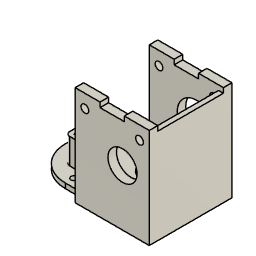
Potentionmeter_Bot (Autodesk Fusion 360 design; units mm, degrees)
Autodesk Fusion 360 part; units mm, degrees
note: some values were not read from the file. Set by a fixed rule: which face or edge a step refers to.
sketch "スケッチ1" plane through (0, 0, 0) normal (0, 0, 1) x (1, 0, 0)
  line L0 (5, -5) -> (-5, -5)
  line L1 (-5, -5) -> (-5, 5)
  line L2 (-5, 5) -> (5, 5)
  line L3 (5, 5) -> (5, -5)
  line L4 (5, -5) -> (-5, 5) construction
  line L5 (-5, -5) -> (5, 5) construction
  line L6 (7, -7) -> (-7, -7)
  line L7 (-7, -7) -> (-7, 7)
  line L8 (-7, 7) -> (7, 7)
  line L9 (7, 7) -> (7, -7)
  line L10 (7, -7) -> (-7, 7) construction
  line L11 (-7, -7) -> (7, 7) construction
  dimension "d1" = 10
  dimension "d2" = 10
  dimension "d3" = 14
  dimension "d4" = 14
  constraint horizontal L0
  constraint perpendicular L0 L1
  constraint parallel L0 L2
  constraint parallel L1 L3
  constraint coincident L4 origin
  constraint coincident L5 origin
  constraint horizontal L6
  constraint perpendicular L6 L7
  constraint parallel L6 L8
  constraint parallel L7 L9
  constraint coincident L10 origin
  constraint coincident L11 origin
  measures "d1" distance of L1.end L2.end
  measures "d2" distance of L0.end L1.end
  measures "d3" distance of L7.end L8.end
  measures "d4" distance of L6.end L7.end
extrude "押し出し1" add sketch "スケッチ1" along normal blind 8 contours L6 L7 L8 L9 picked at (-6.333333, 1.666667) makes body 1
sketch "スケッチ2" plane through (0, 0, 0) normal (0, 0, -1) x (1, 0, 0)
  line L0 (5, -5) -> (-5, -5)
  line L1 (-5, -5) -> (-5, 5)
  line L2 (-5, 5) -> (5, 5)
  line L3 (5, 5) -> (5, -5)
  line L4 (-7, -7) -> (7, -7)
  line L5 (7, -7) -> (7, 7)
  line L6 (7, 7) -> (-7, 7)
  line L7 (-7, 7) -> (-7, -7)
  circle A0 centre (0, 7) radius 7
  circle A1 centre (0, -7) radius 7
  circle A2 centre (7, 0) radius 7
  circle A3 centre (-7, 0) radius 7
  constraint midpoint L6 A0.centre
  constraint coincident L5.end A0
  constraint midpoint L4 A1.centre
  constraint coincident L4.end A1
  constraint midpoint L5 A2.centre
  constraint coincident L4.end A2
  constraint midpoint L7 A3.centre
  constraint coincident L4.start A3
extrude "押し出し2" add sketch "スケッチ2" against normal blind 2 contours L4 A1 | L5 A2 | L7 A3 | L6 A0 picked at (0.519216, -9.274832) picked at (8.528008, 1.763416) picked at (-9.326809, -0.17437) picked at (-0.17437, 9.326809) bodies 1
cylinder "円柱プリミティブ1" cut diameter 2.5 height -14 placed x (0, 0, -1) y (0, 1, 0) z (1, 0, 0) at (7, 0, 5) bodies 1
sketch "スケッチ4" plane through (0, 0, 2) normal (0, 0, 1) x (-1, 0, 0)
  arc A0 (7, 7) -> (-7, 7) centre (0, 7) ccw
  line L0 (-7, 7) -> (7, 7)
  line L1 (0, 7) -> (0, 14)
  circle A1 centre (0, 10.5) radius 1.25
  dimension "d11" = 2.5
  constraint coincident A0.centre L1.start
  constraint midpoint A0 L1.end
  constraint midpoint L1 A1.centre
  measures "d11" diameter of A1
sketch "スケッチ5" plane through (0, 0, 2) normal (0, 0, 1) x (-1, 0, 0)
  arc A0 (7, -7) -> (7, 7) centre (7, 0) ccw
  line L0 (7, 7) -> (7, -7)
  line L1 (7, 0) -> (14, 0)
  circle A1 centre (10.5, 0) radius 1.25
  dimension "d12" = 2.5
  constraint coincident A0.centre L1.start
  constraint midpoint A0 L1.end
  constraint midpoint L1 A1.centre
  measures "d12" diameter of A1
sketch "スケッチ6" plane through (0, 0, 2) normal (0, 0, 1) x (-1, 0, 0)
  arc A0 (-7, -7) -> (7, -7) centre (0, -7) ccw
  line L0 (7, -7) -> (-7, -7)
  line L1 (0, -7) -> (0, -14)
  circle A1 centre (0, -10.5) radius 1.25
  dimension "d13" = 2.5
  constraint coincident A0.centre L1.start
  constraint midpoint A0 L1.end
  constraint midpoint L1 A1.centre
  measures "d13" diameter of A1
sketch "スケッチ7" plane through (0, 0, 2) normal (0, 0, 1) x (-1, 0, 0)
  arc A0 (-7, 7) -> (-7, -7) centre (-7, 0) ccw
  line L0 (-7, -7) -> (-7, 7)
  line L1 (-7, 0) -> (-14, 0)
  circle A1 centre (-10.5, 0) radius 1.25
  dimension "d14" = 2.5
  constraint coincident A0.centre L1.start
  constraint midpoint A0 L1.end
  constraint midpoint L1 A1.centre
  measures "d14" diameter of A1
extrude "押し出し3" cut sketch "スケッチ4" sketch "スケッチ7" sketch "スケッチ6" sketch "スケッチ5" against normal blind 2 contours L1 A1 | L1 A1 picked at (0.272859, 10.814896) picked at (-0.448578, 10.258724) of sketch 2 contours L1 A1 | L1 A1 picked at (-10.25407, 0.510679) picked at (-10.083333, -0.651526) of sketch 3 contours L1 A1 | L1 A1 picked at (-0.644249, -10.180438) picked at (0.17309, -10.120987) of sketch 4 contours L1 A1 | L1 A1 picked at (10.916667, -0.651526) picked at (10.741276, 0.448578) bodies 1
extrude "押し出し4" cut 1 faces at (7.75, 0, 2) along direction (0, 0, -1) blind 2 on bodies 1 bodies 1
sketch "スケッチ8" plane through (0, 0, 0) normal (0, 0, -1) x (1, 0, 0)
  line L0 (7, -7) -> (7, 7)
  arc A0 (7, 7) -> (-7, 7) centre (0, 7) ccw
  arc A1 (-7, 7) -> (-7, -7) centre (-7, 0) ccw
  arc A2 (-7, -7) -> (7, -7) centre (0, -7) ccw
  line L1 (5, -5) -> (-5, -5)
  line L2 (-5, -5) -> (-5, 5)
  line L3 (-5, 5) -> (5, 5)
  line L4 (5, 5) -> (5, -5)
  circle A3 centre (-10.5, 0) radius 1.25
  circle A4 centre (0, 10.5) radius 1.25
  circle A5 centre (0, -10.5) radius 1.25
  line L5 (-10.5, 0) -> (26.5, 0)
  line L6 (26.5, -5) -> (-10.5, -5)
  line L7 (-10.5, -5) -> (-10.5, 5)
  line L8 (-10.5, 5) -> (26.5, 5)
  line L9 (26.5, 5) -> (26.5, -5)
  line L10 (26.5, -5) -> (-10.5, 5) construction
  line L11 (-10.5, -5) -> (26.5, 5) construction
  circle A6 centre (26.5, 0) radius 8
  line L12 (26.5, 5) -> (26.5, 8)
  line L13 (18.5, 0) -> (18.5, 8)
  line L14 (18.5, 8) -> (26.5, 8)
  line L15 (18.5, 0) -> (18.5, -8)
  line L16 (26.5, -5) -> (26.5, -8)
  line L17 (26.5, -8) -> (18.5, -8)
  line L18 (18.5, -8) -> (14.5, -8)
  line L19 (18.5, 8) -> (14.5, 8)
  line L20 (14.5, -8) -> (14.5, 8)
  point P0 (8, 0)
  dimension "d19" = 37
  dimension "d20" = 37
  dimension "d21" = 10
  dimension "d22" = 16
  dimension "d27" = 4
  dimension "d28" = 4
  constraint coincident A3.centre L5.start
  constraint perpendicular L0 L5
  constraint horizontal L6
  constraint perpendicular L6 L7
  constraint parallel L6 L8
  constraint parallel L7 L9
  constraint coincident L10 P0
  constraint coincident L11 P0
  constraint midpoint L5 P0
  constraint coincident L5.end A6.centre
  constraint coincident A6 L12.end
  constraint perpendicular L8 L12
  constraint coincident L5 L13.start
  constraint coincident A6 L13.start
  constraint tangent A6 L13
  constraint perpendicular L13 L14
  constraint tangent A6 L15
  constraint coincident A6 L16.end
  constraint perpendicular L6 L16
  constraint perpendicular L15 L17
  constraint perpendicular L15 L18
  constraint perpendicular L13 L19
  measures "d19" distance of A3.centre L5.end
  measures "d20" distance of L7.end L8.end
  measures "d21" distance of L6.end L7.end
  measures "d22" diameter of A6
  measures "d27" distance of L15.end L18.end
  measures "d28" distance of L13.end L19.end
extrude "押し出し5" add sketch "スケッチ8" against normal blind 11 separate body contours L5 L6 L15 L20 | L6 L15 L18 L20 | L5 L8 L13 L20 | L6 A6 L15 | L6 A6 L15 L17 | L8 L13 L19 L20 | L8 A6 L13 | L8 A6 L13 L14 picked at (15.833333, -1.666667) picked at (15.833333, -6) picked at (15.833333, 1.666667) picked at (19.464588, -4.704603) picked at (19.085001, -6) picked at (17.166667, 6) picked at (19.464588, 4.704603) picked at (19.085001, 6) makes body 2
extrude "押し出し6" add sketch "スケッチ8" against normal blind 2 contours L0 L5 L6 L20 | L0 L5 L8 L20 | L5 L6 L15 L20 | L5 L8 L13 L20 picked at (9.5, -3.333333) picked at (9.5, 3.333333) picked at (15.833333, -1.666667) picked at (15.833333, 1.666667) bodies 1 2
sketch "スケッチ9" plane through (0, 0, 11) normal (0, 0, 1) x (-1, 0, 0)
  line L0 (-14.5, 8) -> (-26.5, 8)
  arc A0 (-26.5, -8) -> (-26.5, 8) centre (-26.5, 0) ccw
  line L1 (-26.5, -8) -> (-14.5, -8)
  line L2 (-14.5, -8) -> (-14.5, 8)
  line L3 (-26.5, 0) -> (-18.5, 0)
  line L4 (-22.5, 0) -> (-22.5, -8)
  line L5 (-22.5, 0) -> (-22.5, 8)
  constraint coincident A0.centre L3.start
  constraint midpoint A0 L3.end
  constraint midpoint L3 L4.start
  constraint coincident L1 L4.end
  constraint perpendicular L1 L4
  constraint coincident L0 L5.end
  constraint perpendicular L0 L5
extrude "押し出し7" cut sketch "スケッチ9" against normal blind 11 contours L0 A0 L5 | A0 L1 L4 picked at (-22.812844, 7.439747) picked at (-22.812844, -7.439747) bodies 1
extrude "押し出し8" add 1 faces at (7, 4.415502, 5.031138) along direction (1, 0, 0) blind 7.5 on bodies 1 bodies 1
extrude "押し出し9" cut 1 faces at (19.833333, -8, 3.666667) along direction (0, 1, 0) blind 1 on bodies 1 bodies 1
extrude "押し出し10" cut 1 faces at (19.833334, 8, 3.666667) along direction (0, -1, 0) blind 1 on bodies 1 bodies 1
sketch "スケッチ10" plane through (0, 0, 11) normal (0, 0, 1) x (-1, 0, 0)
  line L0 (-22.5, -7) -> (-14.5, -7)
  line L1 (-14.5, -7) -> (-14.5, 7)
  line L2 (-14.5, 7) -> (-22.5, 7)
  line L3 (-22.5, 7) -> (-22.5, 6.928203)
  arc A0 (-22.5, -6.928203) -> (-22.5, 6.928203) centre (-26.5, 0) ccw
  line L4 (-22.5, -6.928203) -> (-22.5, -7)
  line L5 (-22.5, -6.928203) -> (-22.5, 6.928203)
  circle A1 centre (-26.5, 0) radius 8.25
  dimension "d37" = 16.5
  constraint concentric A0 A1
  measures "d37" diameter of A1
extrude "押し出し11" cut sketch "スケッチ10" against normal blind 11 contours L0 L2 L3 A0 L4 A1 picked at (-22.048673, -6.727619) bodies 1
extrude "押し出し12" add 1 faces at (14.5, 2.333333, 10) along direction (-1, 0, 0) blind 7.5 on bodies 1 bodies 1
sketch "スケッチ11" plane through (0, -7, 0) normal (0, -1, 0) x (1, 0, 0)
  line L0 (22.133938, 0) -> (22.133938, 11)
  line L1 (22.133938, 11) -> (7, 11)
  line L2 (7, 11) -> (7, 8)
  line L3 (7, 8) -> (-7, 8)
  line L4 (-7, 8) -> (-7, 2)
  line L5 (-7, 2) -> (7, 2)
  line L6 (7, 2) -> (7, 0)
  line L7 (7, 0) -> (22.133938, 0)
  line L8 (7, 11) -> (7, 0)
  constraint coincident L1.end L2.start
  constraint coincident L6.end L7.start
extrude "押し出し13" add sketch "スケッチ11" along normal blind 8 contours L0 L1 L2 L6 L7 L8 picked at (17.089292, 6.333333) bodies 1
sketch "スケッチ12" plane through (0, 7, 0) normal (0, 1, 0) x (-1, 0, 0)
  line L0 (-22.133938, 11) -> (-22.133938, 0)
  line L1 (-22.133938, 0) -> (-7, 0)
  line L2 (-7, 0) -> (-7, 2)
  line L3 (-7, 2) -> (7, 2)
  line L4 (7, 2) -> (7, 8)
  line L5 (7, 8) -> (-7, 8)
  line L6 (-7, 8) -> (-7, 11)
  line L7 (-7, 11) -> (-22.133938, 11)
  line L8 (-7, 11) -> (-7, 0)
  constraint coincident L6.end L7.start
  constraint coincident L1.end L2.start
extrude "押し出し14" add sketch "スケッチ12" along normal blind 8 contours L0 L1 L2 L6 L7 L8 picked at (-17.089292, 6.333333) bodies 1
sketch "スケッチ13" plane through (0, 0, 11) normal (0, 0, 1) x (-1, 0, 0)
  arc A0 (-22.133938, -7) -> (-22.133938, 7) centre (-26.5, 0) ccw
  line L0 (-22.133938, -7) -> (-22.133938, -15)
  line L1 (-22.133938, -15) -> (-7, -15)
  line L2 (-7, -15) -> (-7, 15)
  line L3 (-7, 15) -> (-22.133938, 15)
  line L4 (-22.133938, 15) -> (-22.133938, 7)
  circle A1 centre (-26.5, 0) radius 8.25
  line L5 (-26.5, 0) -> (-22.133938, 0)
  line L6 (-22.133938, 0) -> (-22.133938, -15)
  line L7 (-22.133938, -15) -> (-26.5, -15)
  line L8 (-26.5, -15) -> (-26.5, 0)
  line L9 (-26.5, 0) -> (-22.133938, 0)
  line L10 (-22.133938, 0) -> (-22.133938, 15)
  line L11 (-22.133938, 15) -> (-26.5, 15)
  line L12 (-26.5, 15) -> (-26.5, 0)
  constraint concentric A0 A1
  constraint horizontal L5
  constraint vertical L6
  constraint horizontal L7
  constraint vertical L8
  constraint coincident A0.centre A1.centre
  constraint horizontal L9
  constraint vertical L10
  constraint horizontal L11
  constraint vertical L12
extrude "押し出し15" add sketch "スケッチ13" against normal blind 11 contours L0 A1 L6 L7 L8 | L4 A1 L10 L11 L12 picked at (-24.662481, -12.723316) picked at (-24.662481, 12.723316) bodies 1
sketch "スケッチ14" plane through (0, 0, 11) normal (0, 0, 1) x (-1, 0, 0)
  arc A0 (-26.5, -8.25) -> (-26.5, 8.25) centre (-26.5, 0) ccw
  line L0 (-26.5, -8.25) -> (-26.5, -15)
  line L1 (-26.5, -15) -> (-7, -15)
  line L2 (-7, -15) -> (-7, 15)
  line L3 (-7, 15) -> (-26.5, 15)
  line L4 (-26.5, 15) -> (-26.5, 8.25)
  line L5 (-7, 15) -> (-26.5, 15)
  line L6 (-26.5, 15) -> (-26.5, 17)
  line L7 (-26.5, 17) -> (-7, 17)
  line L8 (-7, 17) -> (-7, 15)
  line L9 (-7, -15) -> (-26.5, -15)
  line L10 (-26.5, -15) -> (-26.5, -17)
  line L11 (-26.5, -17) -> (-7, -17)
  line L12 (-7, -17) -> (-7, -15)
  dimension "d48" = 2
  dimension "d49" = 2
  constraint horizontal L5
  constraint vertical L6
  constraint horizontal L7
  constraint vertical L8
  constraint coincident L2.end L3.start
  constraint horizontal L9
  constraint vertical L10
  constraint horizontal L11
  constraint vertical L12
  constraint coincident L1.end L2.start
  measures "d48" distance of L2.end L7.end
  measures "d49" distance of L1.end L11.end
extrude "押し出し16" add sketch "スケッチ14" along normal blind 2 separate body contours L1 L9 L10 L11 L12 | L3 L5 L6 L7 L8 picked at (-20, -16.333333) picked at (-20, 15.666667) makes body 3 at (20, 15, 11.666667) makes body 4 at (20, -17, 11.666667)
extrude "押し出し17" add 2 faces at (20, -15.666667, 11) (20, 16.333333, 11) along direction (0, 0, -1) blind 11 on bodies 3 4 bodies 1 4 3
extrude "押し出し18" add 1 faces at (20, -15.666667, 13) along direction (0, 0, 1) blind 28 on bodies 1 bodies 1
extrude "押し出し19" add 1 faces at (26.5, -13.416667, 3.666667) along direction (1, 0, 0) blind 11 on bodies 1 bodies 1
extrude "押し出し20" add 1 faces at (26.5, 13.416667, 3.666667) along direction (1, 0, 0) blind 11 on bodies 1 bodies 1
sketch "スケッチ15" plane through (0, -15, 0) normal (0, 1, 0) x (-1, 0, 0)
  line L0 (-37.5, 11) -> (-7, 11)
  line L1 (-7, 11) -> (-7, 41)
  line L2 (-7, 41) -> (-37.5, 41)
  line L3 (-7, 11) -> (-26.5, 11)
  line L4 (-26.5, 11) -> (-26.5, 23)
  line L5 (-26.5, 23) -> (-7, 23)
  line L6 (-7, 23) -> (-7, 11)
  circle A0 centre (-26.5, 23) radius 6
  line L7 (-37.5, 41) -> (-37.5, 11)
  line L8 (-37.5, 11) -> (-7, 11)
  line L9 (-7, 11) -> (-7, 41)
  line L10 (-7, 41) -> (-37.5, 41)
  line L11 (-37.5, 41) -> (-37.5, 11)
  line L12 (-7, 41) -> (-11, 41)
  line L13 (-11, 41) -> (-11, 35.5)
  line L14 (-11, 35.5) -> (-7, 35.5)
  line L15 (-7, 35.5) -> (-7, 41)
  line L16 (-37.5, 41) -> (-33.5, 41)
  line L17 (-33.5, 41) -> (-33.5, 35.5)
  line L18 (-33.5, 35.5) -> (-37.5, 35.5)
  line L19 (-37.5, 35.5) -> (-37.5, 41)
  circle A1 centre (-33.5, 35.5) radius 1.6
  circle A2 centre (-11, 35.5) radius 1.6
  dimension "d56" = 19.5
  dimension "d57" = 12
  dimension "d58" = 12
  dimension "d63" = 4
  dimension "d64" = 5.5
  dimension "d65" = 4
  dimension "d66" = 5.5
  dimension "d67" = 3.2
  dimension "d68" = 3.2
  constraint horizontal L3
  constraint vertical L4
  constraint horizontal L5
  constraint vertical L6
  constraint coincident L0.end L1.start
  constraint coincident L4.end L5.start
  constraint horizontal L12
  constraint vertical L13
  constraint horizontal L14
  constraint vertical L15
  constraint coincident L1.end L2.start
  constraint horizontal L16
  constraint vertical L17
  constraint horizontal L18
  constraint vertical L19
  constraint coincident L2.end L7.start
  constraint coincident L17.end L18.start
  constraint coincident L13.end L14.start
  measures "d56" distance of L0.end L3.end
  measures "d57" distance of L0.end L5.end
  measures "d58" diameter of A0
  measures "d63" distance of L1.end L12.end
  measures "d64" distance of L1.end L14.end
  measures "d65" distance of L2.end L16.end
  measures "d66" distance of L2.end L18.end
  measures "d67" diameter of A1
  measures "d68" diameter of A2
extrude "押し出し21" cut sketch "スケッチ15" against normal blind 2 contours L4 L5 A0 | L4 L5 A0 | L17 L18 A1 | L17 L18 A1 | L13 L14 A2 | L13 L14 A2 picked at (-24.706428, 26.563216) picked at (-22.520357, 22.71537) picked at (-34.351735, 36.137601) picked at (-34.56071, 35.420511) picked at (-9.939106, 35.421744) picked at (-10.066194, 36.009896) bodies 1
sketch "スケッチ16" plane through (0, 0, 11) normal (0, 0, 1) x (-1, 0, 0)
  arc A0 (-26.5, -8.25) -> (-26.5, 8.25) centre (-26.5, 0) ccw
  line L0 (-26.5, -8.25) -> (-37.5, -8.25)
  line L1 (-37.5, -8.25) -> (-37.5, -15)
  line L2 (-37.5, -15) -> (-7, -15)
  line L3 (-7, -15) -> (-7, 15)
  line L4 (-7, 15) -> (-37.5, 15)
  line L5 (-37.5, 15) -> (-37.5, 8.25)
  line L6 (-37.5, 8.25) -> (-26.5, 8.25)
  circle A1 centre (-26.5, 0) radius 8.25
  line L7 (-37.5, -8.25) -> (-37.5, 8.25)
  constraint concentric A0 A1
  constraint coincident L0.end L1.start
  constraint coincident L5.end L6.start
extrude "押し出し22" add sketch "スケッチ16" against normal blind 11 contours L0 L6 A1 L7 picked at (-36.575644, 0.205508) bodies 1
extrude "押し出し23" add 1 faces at (14.5, -0.095795, 5.342047) along direction (-1, 0, 0) blind 9.5 on bodies 1 bodies 1
sketch "スケッチ17" plane through (0, 0, 8) normal (0, 0, 1) x (-1, 0, 0)
  line L0 (-7, 7) -> (-7, -7)
  line L1 (-7, -7) -> (7, -7)
  line L2 (7, -7) -> (7, 7)
  line L3 (7, 7) -> (-7, 7)
  line L4 (5, -5) -> (-5, -5)
  line L5 (-5, -5) -> (-5, 5)
  line L6 (-5, 5) -> (5, 5)
  line L7 (5, 5) -> (5, -5)
  line L8 (-5.25, 5.25) -> (5.25, 5.25)
  line L9 (5.25, 5.25) -> (5.25, -5.25)
  line L10 (5.25, -5.25) -> (-5.25, -5.25)
  line L11 (-5.25, -5.25) -> (-5.25, 5.25)
  line L12 (-5.25, 5.25) -> (5.25, -5.25) construction
  line L13 (5.25, 5.25) -> (-5.25, -5.25) construction
  dimension "d75" = 10.5
  dimension "d76" = 10.5
  constraint horizontal L8
  constraint perpendicular L8 L9
  constraint parallel L8 L10
  constraint parallel L9 L11
  constraint coincident L12 origin
  constraint coincident L13 origin
  measures "d75" distance of L9.end L10.end
  measures "d76" distance of L8.end L9.end
extrude "押し出し24" cut sketch "スケッチ17" against normal blind 8 contours L8 L9 L10 L11 picked at (1.666667, -5.166667) bodies 1
extrude "押し出し25" add 1 faces at (6.416667, -1.75, 8) along direction (0, 0, 1) blind 3 on bodies 1 bodies 1
sketch "スケッチ18" plane through (0, 0, 0) normal (0, 0, -1) x (1, 0, 0)
  line L0 (-5.25, -5.25) -> (-5.25, 5.25)
  line L1 (-5.25, 5.25) -> (5.25, 5.25)
  line L2 (5.25, 5.25) -> (5.25, -5.25)
  line L3 (5.25, -5.25) -> (-5.25, -5.25)
  line L4 (37.5, -17) -> (37.5, 17)
  line L5 (37.5, 17) -> (7, 17)
  line L6 (7, 17) -> (7, 7)
  arc A0 (7, 7) -> (-7, 7) centre (0, 7) ccw
  arc A1 (-7, 7) -> (-7, -7) centre (-7, 0) ccw
  arc A2 (-7, -7) -> (7, -7) centre (0, -7) ccw
  line L7 (7, -7) -> (7, -17)
  line L8 (7, -17) -> (37.5, -17)
  circle A3 centre (26.5, 0) radius 8.25
  circle A4 centre (-10.5, 0) radius 1.25
  circle A5 centre (0, 10.5) radius 1.25
  circle A6 centre (0, -10.5) radius 1.25
  line L9 (0, 14) -> (7, 14)
  line L10 (0, -14) -> (7, -14)
  constraint midpoint A0 L9.start
  constraint coincident L6 L9.end
  constraint tangent A0 L9
  constraint perpendicular L6 L9
  constraint midpoint A2 L10.start
  constraint tangent A2 L10
  constraint perpendicular L6 L10
extrude "押し出し26" add sketch "スケッチ18" against normal blind 2 contours A2 L7 L10 | L6 A0 L9 picked at (5.624757, -12.624757) picked at (5.624757, 12.624757) bodies 1
extrude "押し出し27" add 1 faces at (17.166667, 15.666667, 13) along direction (0, 0, 1) blind 28 on bodies 1 bodies 1
sketch "スケッチ19" plane through (0, 0, 41) normal (0, 0, 1) x (-1, 0, 0)
  line L0 (-7, -17) -> (-7, -15)
  line L1 (-7, -15) -> (-37.5, -15)
  line L2 (-37.5, -15) -> (-37.5, -17)
  line L3 (-37.5, -17) -> (-7, -17)
  line L4 (-22.25, -17) -> (-22.25, -15)
  line L5 (-27.25, -15) -> (-17.25, -15)
  line L6 (-17.25, -15) -> (-17.25, -17)
  line L7 (-17.25, -17) -> (-27.25, -17)
  line L8 (-27.25, -17) -> (-27.25, -15)
  line L9 (-27.25, -15) -> (-17.25, -17) construction
  line L10 (-17.25, -15) -> (-27.25, -17) construction
  point P0 (-22.25, -16)
  dimension "d85" = 10
  constraint midpoint L3 L4.start
  constraint midpoint L1 L4.end
  constraint horizontal L5
  constraint perpendicular L5 L6
  constraint parallel L5 L7
  constraint parallel L6 L8
  constraint coincident L9 P0
  constraint coincident L10 P0
  constraint midpoint L4 P0
  measures "d85" distance of L6.end L7.end
sketch "スケッチ20" plane through (0, 0, 41) normal (0, 0, 1) x (-1, 0, 0)
  line L0 (-7, 17) -> (-37.5, 17)
  line L1 (-37.5, 17) -> (-37.5, 15)
  line L2 (-37.5, 15) -> (-7, 15)
  line L3 (-7, 15) -> (-7, 17)
  line L4 (-22.25, 15) -> (-22.25, 17)
  line L5 (-27.25, 17) -> (-17.25, 17)
  line L6 (-17.25, 17) -> (-17.25, 15)
  line L7 (-17.25, 15) -> (-27.25, 15)
  line L8 (-27.25, 15) -> (-27.25, 17)
  line L9 (-27.25, 17) -> (-17.25, 15) construction
  line L10 (-17.25, 17) -> (-27.25, 15) construction
  point P0 (-22.25, 16)
  dimension "d86" = 10
  constraint midpoint L2 L4.start
  constraint midpoint L0 L4.end
  constraint horizontal L5
  constraint perpendicular L5 L6
  constraint parallel L5 L7
  constraint parallel L6 L8
  constraint coincident L9 P0
  constraint coincident L10 P0
  constraint midpoint L4 P0
  measures "d86" distance of L6.end L7.end
extrude "押し出し28" cut sketch "スケッチ20" sketch "スケッチ19" against normal blind 2 contours L0 L2 L4 L5 L6 L7 | L0 L2 L4 L5 L7 L8 picked at (-20.583333, 16.333333) picked at (-23.916667, 15.666667) of sketch 2 contours L1 L3 L4 L5 L6 L7 | L1 L3 L4 L5 L7 L8 picked at (-18.916667, -16.333333) picked at (-23.916667, -16.333333) bodies 1
extrude "押し出し29" add 1 faces at (12.714656, -15, 22.646705) along direction (0, 1, 0) blind 1.5 on bodies 1 bodies 1
extrude "押し出し30" add 1 faces at (20.583333, 15, 20.333333) along direction (0, -1, 0) blind 1.5 on bodies 1 bodies 1
sketch "スケッチ21" plane through (0, 13.5, 0) normal (0, -1, 0) x (1, 0, 0)
  line L0 (27.25, 41) -> (27.25, 39)
  line L1 (27.25, 39) -> (17.25, 39)
  line L2 (17.25, 39) -> (17.25, 41)
  line L3 (17.25, 41) -> (7, 41)
  line L4 (7, 41) -> (7, 11)
  line L5 (7, 11) -> (37.5, 11)
  line L6 (37.5, 11) -> (37.5, 41)
  line L7 (37.5, 41) -> (27.25, 41)
  line L8 (37.5, 11) -> (26.5, 11)
  line L9 (26.5, 11) -> (26.5, 23)
  line L10 (26.5, 23) -> (37.5, 23)
  line L11 (37.5, 23) -> (37.5, 11)
  circle A0 centre (26.5, 23) radius 8
  dimension "d93" = 11
  dimension "d94" = 12
  dimension "d95" = 16
  constraint horizontal L8
  constraint vertical L9
  constraint horizontal L10
  constraint vertical L11
  constraint coincident L5.end L6.start
  constraint coincident L9.end L10.start
  measures "d93" distance of L5.end L8.end
  measures "d94" distance of L5.end L10.end
  measures "d95" diameter of A0
extrude "押し出し31" cut sketch "スケッチ21" against normal blind 3.5 contours L9 L10 A0 | L9 L10 A0 picked at (31.484333, 21.14094) picked at (26.108719, 17.695529) bodies 1
sketch "スケッチ22" plane through (0, 17, 0) normal (0, 1, 0) x (-1, 0, 0)
  circle A0 centre (-26.5, 23) radius 8
  line L0 (-27.25, 39) -> (-27.25, 41)
  line L1 (-27.25, 41) -> (-37.5, 41)
  line L2 (-37.5, 41) -> (-37.5, 0)
  line L3 (-37.5, 0) -> (-7, 0)
  line L4 (-7, 0) -> (-7, 41)
  line L5 (-7, 41) -> (-17.25, 41)
  line L6 (-17.25, 41) -> (-17.25, 39)
  line L7 (-17.25, 39) -> (-27.25, 39)
  line L8 (-37.5, 41) -> (-33.5, 41)
  line L9 (-33.5, 41) -> (-33.5, 35.5)
  line L10 (-33.5, 35.5) -> (-37.5, 35.5)
  line L11 (-37.5, 35.5) -> (-37.5, 41)
  line L12 (-7, 41) -> (-11, 41)
  line L13 (-11, 41) -> (-11, 35.5)
  line L14 (-11, 35.5) -> (-7, 35.5)
  line L15 (-7, 35.5) -> (-7, 41)
  circle A1 centre (-33.5, 35.5) radius 1.6
  circle A2 centre (-11, 35.5) radius 1.6
  dimension "d98" = 4
  dimension "d99" = 5.5
  dimension "d100" = 4
  dimension "d101" = 5.5
  dimension "d102" = 3.2
  dimension "d103" = 3.2
  constraint horizontal L8
  constraint vertical L9
  constraint horizontal L10
  constraint vertical L11
  constraint coincident L1.end L2.start
  constraint horizontal L12
  constraint vertical L13
  constraint horizontal L14
  constraint vertical L15
  constraint coincident L4.end L5.start
  constraint coincident L9.end L10.start
  constraint coincident L13.end L14.start
  measures "d98" distance of L1.end L8.end
  measures "d99" distance of L1.end L10.end
  measures "d100" distance of L4.end L12.end
  measures "d101" distance of L4.end L14.end
  measures "d102" diameter of A1
  measures "d103" diameter of A2
extrude "押し出し32" cut sketch "スケッチ22" against normal blind 4.5 contours L9 L10 A1 | L9 L10 A1 | L13 L14 A2 | L13 L14 A2 picked at (-34.56071, 35.420511) picked at (-34.351735, 36.137601) picked at (-10.066194, 36.009896) picked at (-9.939106, 35.421744) bodies 1
sketch "スケッチ23" plane through (0, 0, 0) normal (0, 0, -1) x (1, 0, 0)
  line L0 (-5.25, -5.25) -> (-5.25, 5.25)
  line L1 (-5.25, 5.25) -> (5.25, 5.25)
  line L2 (5.25, 5.25) -> (5.25, -5.25)
  line L3 (5.25, -5.25) -> (-5.25, -5.25)
  line L4 (37.5, -17) -> (37.5, 17)
  line L5 (37.5, 17) -> (7, 17)
  line L6 (7, 17) -> (7, 14)
  line L7 (7, 14) -> (0, 14)
  arc A0 (0, 14) -> (-7, 7) centre (0, 7) ccw
  arc A1 (-7, 7) -> (-7, -7) centre (-7, 0) ccw
  arc A2 (-7, -7) -> (0, -14) centre (0, -7) ccw
  line L8 (0, -14) -> (7, -14)
  line L9 (7, -14) -> (7, -17)
  line L10 (7, -17) -> (37.5, -17)
  circle A3 centre (26.5, 0) radius 8.25
  circle A4 centre (-10.5, 0) radius 1.25
  circle A5 centre (0, 10.5) radius 1.25
  circle A6 centre (0, -10.5) radius 1.25
  line L11 (-5.25, 5.25) -> (5.25, -5.25)
  line L12 (5.25, 5.25) -> (-5.25, -5.25)
  circle A7 centre (0, 0) radius 14
  constraint coincident L0.end L1.start
  constraint coincident L2.end L3.start
  constraint coincident L1.end L2.start
  constraint coincident L0.start L3.end
  constraint coincident A7.centre origin
  constraint tangent A1 A7
extrude "押し出し33" add sketch "スケッチ23" against normal blind 2 contours A1 A2 A7 | A0 A1 A7 picked at (-9.248249, -8.892431) picked at (-8.892431, 9.248249) bodies 1
fillet "フィレット1" radius 1.75 2 edges at (-7, -7, 6.5) (-7, 7, 6.5) on bodies 1
extrude "押し出し34" add 1 faces at (9.583624, 0.039981, 11) along direction (0, 0, 1) blind 1.5 on bodies 1 bodies 1
sketch "スケッチ24" plane through (0, 0, 12.5) normal (0, 0, 1) x (-1, 0, 0)
  arc A0 (5.25, -7) -> (7, -5.25) centre (5.25, -5.25) ccw
  line L0 (7, -5.25) -> (7, 5.25)
  arc A1 (7, 5.25) -> (5.25, 7) centre (5.25, 5.25) ccw
  line L1 (5.25, 7) -> (-7, 7)
  line L2 (-7, 7) -> (-7, 13.5)
  line L3 (-7, 13.5) -> (-37.5, 13.5)
  line L4 (-37.5, 13.5) -> (-37.5, -13.5)
  line L5 (-37.5, -13.5) -> (-7, -13.5)
  line L6 (-7, -13.5) -> (-7, -7)
  line L7 (-7, -7) -> (5.25, -7)
  circle A2 centre (-26.5, 0) radius 8.25
  line L8 (5.25, 5.25) -> (5.25, -5.25)
  line L9 (5.25, -5.25) -> (-5.25, -5.25)
  line L10 (-5.25, -5.25) -> (-5.25, 5.25)
  line L11 (-5.25, 5.25) -> (5.25, 5.25)
  line L12 (-37.5, -13.5) -> (-35.5, -13.5)
  line L13 (-35.5, -13.5) -> (-35.5, 13.5)
  line L14 (-35.5, 13.5) -> (-37.5, 13.5)
  line L15 (-37.5, 13.5) -> (-37.5, -13.5)
  dimension "d112" = 2
  constraint horizontal L12
  constraint vertical L13
  constraint horizontal L14
  constraint vertical L15
  constraint coincident L4.end L5.start
  measures "d112" distance of L4.end L12.end
extrude "押し出し35" add sketch "スケッチ24" along normal blind 26.5 contours L3 L4 L5 L12 L13 L14 L15 picked at (-36.166667, -4.5) bodies 1
